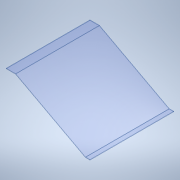
# Autodesk Inventor part: Bottom Lexan Shield for Balls
Saved by Autodesk Inventor 2021.1 (Build 251245000, 245)
## iProperties
Created: 2021-02-23
Part Number: Bottom Lexan Shield for Balls
Material: Polycarbonate, Clear
Document SubType Name: Modeling
Designer: aidan
Density: 1.2 g/cm^3
Appearance: Tropical Blue
Author: aidan
Autodesk Inventor part; units mm, degrees
ref_plane "YZ Plane" through (0, 0, 0) normal (1, 0, 0) x (0, 1, 0)
ref_plane "XZ Plane" through (0, 0, 0) normal (0, 1, 0) x (-1, 0, 0)
ref_plane "XY Plane" through (0, 0, 0) normal (0, 0, 1) x (1, 0, 0)
sketch "Sketch1" plane through (0, 0, 0) normal (0, 0, 1) x (1, 0, 0)
  line L0 (0, 0) -> (-25.4, 0)
  line L1 (-25.4, 0) -> (-406.4, 203.2)
  line L2 (-406.4, 203.2) -> (-457.2, 203.2)
  line L3 (-457.2, 203.2) -> (-457.2, 206.1972)
  line L4 (-457.2, 206.1972) -> (-405.6507, 206.1972)
  line L5 (-405.6507, 206.1972) -> (-24.6507, 2.9972)
  line L6 (-24.6507, 2.9972) -> (0, 2.9972)
  line L7 (0, 2.9972) -> (0, 0)
  line L8 (-406.4, 203.2) -> (-405.6507, 206.1972) construction
  line L9 (-24.6507, 2.9972) -> (-25.4, 0) construction
  line L10 (0, 0) -> (-457.2, 0) construction
  line L11 (-457.2, 0) -> (-457.2, 206.1972) construction
  line L12 (-457.2, 206.1972) -> (0, 206.1972) construction
  line L13 (0, 206.1972) -> (0, 0) construction
  line L14 (-406.4, 203.2) -> (-449.1958, 32.0169) construction
  dimension "d0" = 2.9972
  dimension "d1" = 2.9972
  dimension "d2" = 381
  dimension "d3" = 203.2
  dimension "d5" = 50.8
  dimension "d6" = 25.4
  dimension "d7" = 151.928
  constraints: 30 end point, 5 parallel, 4 perpendicular, 2 horizontal, 1 collinear, 1 other
  measures "d0" distance between parallel lines of L4 L2
  measures "d1" distance of L6.end L0.start
  measures "d2" horizontal distance of L0.end L1.end
  measures "d3" distance between parallel lines of L0 L2
  measures "d5" distance of L1.end L2.end
  measures "d6" distance of L0.start L0.end
  measures "d7" angle of L1 L2
extrude "Extrusion1" add sketch "Sketch1" along normal blind 558.8
sketch "Sketch2" plane through (0, 0, 558.8) normal (0, 0, 1) x (1, 0, 0)
  line L0 (-25.4, 0) -> (0, 0) projected
  line L1 (0, 0) -> (-25.4, 0)
  line L2 (-457.2, 203.2) -> (-406.4, 203.2) projected
  line L3 (-25.4, 0) -> (-406.4, 203.2)
  line L4 (-406.4, 203.2) -> (-457.2, 203.2)
  line L5 (-457.2, 206.1972) -> (-457.2, 203.2) projected
  line L6 (-457.2, 203.2) -> (-457.2, 206.1972)
  line L7 (-24.6507, 2.9972) -> (-405.6507, 206.1972) projected
  line L8 (-457.2, 206.1972) -> (-405.6507, 206.1972)
  line L9 (-405.6507, 206.1972) -> (-24.6507, 2.9972)
  line L10 (-24.6507, 2.9972) -> (0, 2.9972)
  line L11 (0, 2.9972) -> (0, 0)
  constraints: 16 end point, 3 collinear, 3 perpendicular, 1 parallel
extrude "Extrusion2" cut sketch "Sketch2" against normal blind 50.8
sketch "Sketch3" plane through (0, 0, 0) normal (0, 0, -1) x (-1, 0, 0)
  line L0 (406.4, 203.2) -> (25.4, 0) projected
  line L1 (0, 0) -> (25.4, 0)
  line L2 (25.4, 0) -> (406.4, 203.2)
  line L3 (457.2, 203.2) -> (406.4, 203.2) projected
  line L4 (406.4, 203.2) -> (457.2, 203.2)
  line L5 (457.2, 206.1972) -> (457.2, 203.2) projected
  line L6 (457.2, 203.2) -> (457.2, 206.1972)
  line L7 (405.6507, 206.1972) -> (457.2, 206.1972) projected
  line L8 (457.2, 206.1972) -> (405.6507, 206.1972)
  line L9 (24.6507, 2.9972) -> (405.6507, 206.1972) projected
  line L10 (405.6507, 206.1972) -> (24.6507, 2.9972)
  line L11 (0, 2.9972) -> (24.6507, 2.9972) projected
  line L12 (24.6507, 2.9972) -> (0, 2.9972)
  line L13 (0, 0) -> (0, 2.9972) projected
  line L14 (0, 2.9972) -> (0, 0)
  constraints: 16 end point, 3 collinear, 3 perpendicular, 1 horizontal, 1 parallel
extrude "Extrusion3" cut sketch "Sketch3" against normal blind 50.8
body "Solid1"
